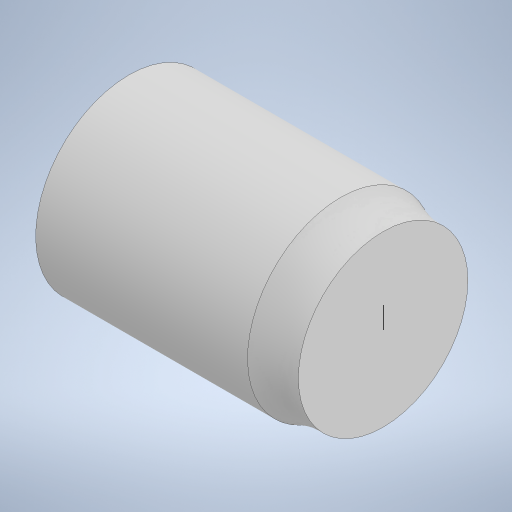
# Autodesk Inventor part: Pieza2_Lab062
Saved by Autodesk Inventor 2024 (Build 280153000, 153)
## iProperties
Created: 2024-02-06
Part Number: Pieza2_Lab062
Material: Genérico
Document SubType Name: Modeling
Designer: pazjo
Density: 1 g/cm^3
Appearance: Valor por defecto
Author: pazjo
Autodesk Inventor part; units mm, degrees
ref_plane "XZ Plane" through (0, 0, 0) normal (0, 1, 0) x (-1, 0, 0)
sketch "Boceto1" plane through (0, 0, 0) normal (0, 0, 1) x (1, 0, 0)
  line L0 (0, 0) -> (0, 200)
  arc A0 (-100, 220) -> (0, 200) centre (-9.4551, 412.7246) ccw
  line L1 (-100, 220) -> (-600, 220)
  line L2 (0, 0) -> (-500, 0)
  line L3 (-600, 220) -> (-600, 0)
  line L4 (-600, 0) -> (0, 0)
  constraints: 10 end point, 2 horizontal, 2 point on circle, 2 vertical, 1 centre point, 1 collinear
revolve "Revolución1" add sketch "Boceto1" angle 360 about axis through (-600, 0, 0) along (1, 0, 0)
ref_plane "Plano de trabajo1" through (0, 0, 200) normal (0, 0, 1) x (1, 0, 0)
ref_plane "Plano de trabajo2" through (210, 0, 0) normal (1, 0, 0) x (0, 1, 0)
sketch "Boceto2" plane through (0, 0, 0) normal (1, 0, 0) x (0, 1, 0)
  line L0 (0, 0) -> (50, 0)
  line L1 (0, 0) -> (50, 0)
  constraints: 4 end point, 2 horizontal
